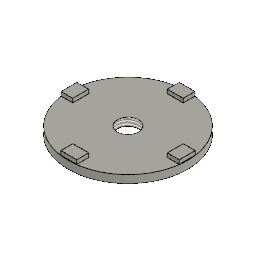
wheel v6 (Autodesk Fusion 360 design; units mm, degrees)
Autodesk Fusion 360 part; units mm, degrees
sketch "wheel" plane through (0, 0, 0) normal (0, 0, 1) x (1, 0, 0)
  circle A0 centre (0, 0) radius 75
  dimension "d1" = 150
  constraint coincident A0.centre origin
  measures "d1" diameter of A0
extrude "Extrude1" add sketch "wheel" along normal blind 10 makes body 1
hole "Hole1" at (0, 0, 10) direction (0, 0, -1) diameter 30 depth 35 tip angle 118 bodies 1
thread "Thread1" "ISO Metric profile 30.0 M30x3.5 6H" major diameter 30.3925 minor diameter 26.491 pitch 3.5 angle 60 resizes the face on face at (0.7477, -14.9814, 6.6667) on bodies 1
ref_plane "WorkPlane1" through (0, 0, 10.25) normal (0, 0, 1) x (1, 0, 0)
sketch "connection block" plane through (0, 0, 10.25) normal (0, 0, 1) x (1, 0, 0)
  circle A0 centre (0, 0) radius 75
  line L0 (-10, 74.3303) -> (10, 74.3303)
  line L1 (10, 59.3303) -> (-10, 59.3303)
  line L2 (-10, 59.3303) -> (-10, 74.3303)
  line L3 (10, 74.3303) -> (10, 59.3303)
  line L4 (-59.3303, -10) -> (-74.3303, -10)
  line L5 (-59.3303, 10) -> (-59.3303, -10)
  line L6 (-74.3303, 10) -> (-59.3303, 10)
  line L7 (-74.3303, -10) -> (-74.3303, 10)
  line L8 (10, -59.3303) -> (10, -74.3303)
  line L9 (-10, -59.3303) -> (10, -59.3303)
  line L10 (-10, -74.3303) -> (-10, -59.3303)
  line L11 (10, -74.3303) -> (-10, -74.3303)
  line L12 (59.3303, 10) -> (74.3303, 10)
  line L13 (59.3303, -10) -> (59.3303, 10)
  line L14 (74.3303, -10) -> (59.3303, -10)
  line L15 (74.3303, 10) -> (74.3303, -10)
  point P0 (-10, 74.3303)
  point P1 (10, 74.3303)
  point P2 (10, 59.3303)
  point P3 (-9.0313, 59.3303)
  dimension "d8" = 20
  dimension "d9" = 15
  dimension "d11" = 360
  constraint coincident P0 A0
  constraint coincident A0 P1
  constraint horizontal P0 L0.end
  constraint vertical P1 P2
  constraint horizontal P2 P3
  constraint coincident P0 L0.start
  constraint coincident P1 L0.end
  constraint coincident P2 L1.start
  constraint parallel L0 L1
  constraint perpendicular L1 L2
  constraint perpendicular L1 L3
  measures "d8" distance of P0 P1
  measures "d9" distance of P1 P2
extrude "Extrude2" add sketch "connection block" along normal blind 5 separate body contours L12 L13 L14 L15 | L0 L1 L2 L3 | L8 L9 L10 L11 | L4 L5 L6 L7 makes body 2 at (69.3303, -3.3333, 10.25) makes body 3 at (3.3333, 69.3303, 10.25) makes body 4 at (-64.3303, 3.3333, 10.25) makes body 5 at (-3.3333, -69.3303, 10.25)
